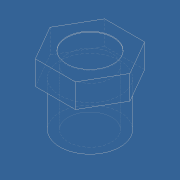
# Autodesk Inventor part: 9833K21
Saved by Autodesk Inventor 2012 SP2 (Build 160219200, 219)
## iProperties
Created: 2012-07-03
Part Number: 9833K21
Material: BRONZE, SAE 841
Description: Breather Vent 1/8 NPT Male, 2 Max SCFM, 7/16" Height
Vendor: MCMASTER
Document SubType Name: Modeling
Designer: JORDANJ
Density: 6.6 g/cm^3
Mass: 3.46355 g
Surface Area: 7.78196 cm^2
Volume: 0.52478 cm^3
RuleStatus: InUse
AfterDocSave0: file://Part Number Cleaner
DESIGN DEPARTMENT: HHMI: JFRC - ID&F
ALTERED ITEM PART NUMBER: N/A
ALTERED ITEM VENDOR: N/A
ALTERED ITEM DESCRIPTION: N/A
Revision Number: 0
Autodesk Inventor part; units mm, degrees
ref_plane "YZ Plane" through (0, 0, 0) normal (1, 0, 0) x (0, 1, 0)
ref_plane "XZ Plane" through (0, 0, 0) normal (0, 1, 0) x (-1, 0, 0)
ref_plane "XY Plane" through (0, 0, 0) normal (0, 0, 1) x (1, 0, 0)
sketch "Sketch1" plane through (0, 0, 0) normal (0, 0, 1) x (1, 0, 0)
  line L0 (0, 0) -> (4.445, 0)
  line L1 (4.445, 0) -> (4.445, 7.2771)
  line L2 (4.445, 7.2771) -> (6.5111, 7.2771)
  line L3 (6.5111, 7.2771) -> (6.5111, 11.176)
  line L4 (6.5111, 11.176) -> (0, 11.176)
  line L5 (0, 11.176) -> (0, 0)
  line L6 (6.5111, 11.176) -> (3.2556, 5.5372) construction
  line L7 (3.2556, 5.5372) -> (-3.2556, 5.5372) construction
  line L8 (-3.2556, 5.5372) -> (-6.5111, 11.176) construction
  line L9 (-6.5111, 11.176) -> (-3.2556, 16.8148) construction
  line L10 (-3.2556, 16.8148) -> (3.2556, 16.8148) construction
  line L11 (3.2556, 16.8148) -> (6.5111, 11.176) construction
  line L12 (3.81, 11.176) -> (3.81, 11.049)
  line L13 (3.81, 11.049) -> (0, 11.049)
  line L14 (3.5179, 0) -> (3.5179, 9.017)
  line L15 (3.5179, 9.017) -> (0, 9.017)
  dimension "d0" = 8.89
  dimension "d2" = 3.8989
  dimension "d3" = 11.2776
  dimension "d7" = 11.176
  dimension "d8" = 7.62
  dimension "d9" = 0.127
  dimension "d10" = 7.0358
  dimension "d11" = 9.017
  constraints: 32 end point, 5 horizontal, 5 vertical, 4 point on line, 1 coincident, 13 other
  measures "d0" diameter of L1 L5
  measures "d2" distance of L2.end L3.end
  measures "d3" distance between parallel lines of L8 L11
  measures "d7" distance between parallel lines of L0 L4
  measures "d8" diameter of L12 L5
  measures "d9" distance between parallel lines of L4 L13
  measures "d10" diameter of L14 L5
  measures "d11" distance of L14.start L14.end
revolve "Revolution1" add sketch "Sketch1" angle 360 about axis through (0, 11.176, 0) along (0, -1, 0) contours L14 L15 L5 L13 L12 L4 L3 L2 L1 L0
sketch "Sketch2" plane through (0, 11.176, 0) normal (0, 1, 0) x (1, 0, 0)
  line L0 (6.5111, 0) -> (3.2556, -5.6388)
  line L1 (3.2556, -5.6388) -> (-3.2556, -5.6388)
  line L2 (-3.2556, -5.6388) -> (-6.5111, 0)
  line L3 (-6.5111, 0) -> (-3.2556, 5.6388)
  line L4 (-3.2556, 5.6388) -> (3.2556, 5.6388)
  line L5 (3.2556, 5.6388) -> (6.5111, 0)
  circle A0 centre (0, 0) radius 6.5111 projected
  constraints: 12 end point, 1 coincident, 1 horizontal, 1 horizontal alignment, 14 other
extrude "Extrusion1" cut sketch "Sketch2" against normal through all contours A0 L0 | L5 A0 | A0 L1 | L4 A0 | A0 L2 | L3 A0
thread "Thread1" size "1/8" designation "1/8 - 27 NPT" standard "NPT" length 9.9568
body "Solid1"
